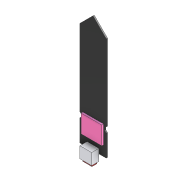
# Autodesk Inventor part: CSM_Sensor_Dummy
Saved by Autodesk Inventor 2020 (Build 240168000, 168)
## iProperties
Created: 2020-08-23
Part Number: CSM_Sensor_Dummy
Material: Generisch
Document SubType Name: Modeling
Designer: uhlma
Density: 1 g/cm^3
Appearance: Glänzend - Schwarz
Author: uhlma
Autodesk Inventor part; units mm, degrees
ref_plane "YZ Plane" through (0, 0, 0) normal (1, 0, 0) x (0, 1, 0)
ref_plane "XZ Plane" through (0, 0, 0) normal (0, 1, 0) x (-1, 0, 0)
ref_plane "XY Plane" through (0, 0, 0) normal (0, 0, 1) x (1, 0, 0)
sketch "Skizze1" plane through (0, 0, 0) normal (0, 0, 1) x (1, 0, 0)
  line L0 (11, -43) -> (-11, -43)
  line L1 (-11, -43) -> (-11, 43)
  line L2 (11, 43) -> (11, -43)
  line L3 (11, -43) -> (-11, 43) construction
  line L4 (-11, -43) -> (11, 43) construction
  line L5 (-11, 43) -> (0, 54)
  line L6 (0, 54) -> (11, 43)
  point P0 (0, 0)
  point P1 (0, 0)
  dimension "d0" = 22
  dimension "d1" = 86
  dimension "d2" = 97
  constraints: 14 end point, 3 midpoint, 1 horizontal, 1 horizontal alignment, 1 parallel, 1 perpendicular, 1 vertical alignment
  measures "d0" distance of L0.start L0.end
  measures "d1" distance of L2.start L0.start
  measures "d2" distance from line of L0 L5.end
extrude "Extrusion1" add sketch "Skizze1" along normal mid plane 1
sketch "Skizze2" plane through (0, 0, 0.5) normal (0, 0, 1) x (1, 0, 0)
  line L0 (-11, -20.5) -> (-9.6, -21.75)
  line L1 (-9.6, -21.75) -> (-9.6, -23.75)
  line L2 (-9.6, -23.75) -> (-11, -25)
  line L3 (-11, -25) -> (-11, -20.5)
  line L4 (-11, 43) -> (-11, -43) projected
  point P0 (0, 0)
  point P1 (-11, -22.75)
  point P2 (-9.6, -22.75)
  dimension "d5" = 1.4
  dimension "d6" = 18
  dimension "d7" = 22.5
  dimension "d8" = 2
  constraints: 8 end point, 2 midpoint, 1 collinear, 1 horizontal alignment, 1 parallel, 1 vertical
  measures "d5" distance between parallel lines of L1 L4
  measures "d6" distance of L4.end L2.end
  measures "d7" distance of L4.end L0.start
  measures "d8" distance of L0.end L1.end
extrude "Extrusion2" cut sketch "Skizze2" against normal blind 1
mirror "Spiegeln1" about plane through (0, 0, 0) normal (1, 0, 0) of "Extrusion2"
sketch "Skizze3" plane through (0, 0, 0.5) normal (0, 0, 1) x (1, 0, 0)
  line L0 (-4.9, -39) -> (4.9, -39)
  line L1 (4.9, -39) -> (4.9, -48.4)
  line L2 (4.9, -48.4) -> (-4.9, -48.4)
  line L3 (-4.9, -48.4) -> (-4.9, -39)
  line L4 (-11, -43) -> (11, -43) projected
  point P0 (0, 0)
  point P1 (0, -39)
  point P2 (0, -43)
  dimension "d11" = 9.4
  dimension "d12" = 9.8
  dimension "d13" = 5.4
  constraints: 8 end point, 2 midpoint, 2 parallel, 1 horizontal, 1 perpendicular, 1 vertical alignment
  measures "d11" distance of L0.end L1.end
  measures "d12" distance of L1.end L2.end
  measures "d13" distance between parallel lines of L4 L2
extrude "Extrusion3" add sketch "Skizze3" along normal blind 6
sketch "Skizze4" plane through (0, 0, 0.5) normal (0, 0, 1) x (1, 0, 0)
  line L0 (-8.4, -19.5) -> (8.8, -19.5)
  line L1 (8.8, -19.5) -> (8.8, -34.5)
  line L2 (8.8, -34.5) -> (-8.4, -34.5)
  line L3 (-8.4, -34.5) -> (-8.4, -19.5)
  line L4 (4.9, -43) -> (11, -43) projected
  line L5 (11, -43) -> (11, -25) projected
  line L6 (-11, -25) -> (-11, -43) projected
  point P0 (0, 0)
  dimension "d16" = 23.5
  dimension "d19" = 8.5
  dimension "d20" = 2.2
  dimension "d21" = 2.6
  constraints: 8 end point, 2 parallel, 1 horizontal, 1 perpendicular
  measures "d16" distance between parallel lines of L4 L0
  measures "d19" distance between parallel lines of L4 L2
  measures "d20" distance between parallel lines of L5 L1
  measures "d21" distance between parallel lines of L6 L3
extrude "Extrusion4" add sketch "Skizze4" along normal blind 1.5
sketch "Skizze5" plane through (-4.9, -48.4, 0.5) normal (0, -1, 0) x (1, 0, 0)
  line L0 (1.0328, 4.6703) -> (8.6704, 4.6703)
  line L1 (8.6704, 4.6703) -> (8.6704, 0.6911)
  line L2 (8.6704, 0.6911) -> (1.0328, 0.6911)
  line L3 (1.0328, 0.6911) -> (1.0328, 4.6703)
  point P0 (4.9, -0.5)
  constraints: 8 end point, 2 parallel, 1 horizontal, 1 perpendicular
extrude "Extrusion5" add sketch "Skizze5" along normal blind 2
